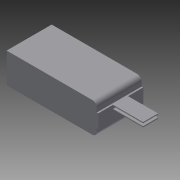
# Autodesk Inventor part: Limit Switch Container
Saved by Autodesk Inventor 2015 (Build 190159000, 159)
## iProperties
Created: 2015-01-10
Part Number: Limit Switch Container
Material: Generic
Document SubType Name: Modeling
Designer: harrykuperstein
Density: 1 g/cm^3
Appearance: Default
Author: harrykuperstein
Autodesk Inventor part; units mm, degrees
ref_plane "YZ Plane" through (0, 0, 0) normal (1, 0, 0) x (0, 1, 0)
ref_plane "XZ Plane" through (0, 0, 0) normal (0, 1, 0) x (-1, 0, 0)
ref_plane "XY Plane" through (0, 0, 0) normal (0, 0, 1) x (1, 0, 0)
sketch "Sketch1" plane through (0, 0, 0) normal (0, 1, 0) x (-1, 0, 0)
  line L0 (0, 0) -> (-30, 0)
  line L1 (-30, 0) -> (-30, -15)
  line L2 (-30, -15) -> (0, -15)
  line L3 (0, -15) -> (0, 0)
  dimension "d0" = 30
  dimension "d1" = 15
  constraints: 8 end point, 2 parallel, 1 horizontal, 1 perpendicular
  measures "d0" distance of L2.end L1.end
  measures "d1" distance of L1.end L0.end
extrude "Extrusion1" add sketch "Sketch1" along normal blind 10
fillet "Fillet1" radius 1.5 1 edges at (30, 10, -7.5)
fillet "Fillet2" radius 1.5 1 edges at (30, 0, -7.5)
fillet "Fillet3" radius 0.5 1 edges at (0, 0, -7.5)
sketch "Sketch2" plane through (30, 8.5, 0) normal (1, 0, 0) x (0, 0, -1)
  line L0 (0, 0) -> (15, 0)
  line L1 (15, 0) -> (0, 0)
  line L2 (15, -7) -> (0, -7) projected
  line L3 (0, -7) -> (0, -6)
  line L4 (0, -6) -> (15, -6)
  line L5 (15, -6) -> (15, -1.3619)
  line L6 (15, -1.3619) -> (0, -1.3619)
  line L7 (0, -1.3619) -> (0, -6)
  point P0 (0, -8.5)
  dimension "d7" = 1
  constraints: 14 end point, 3 horizontal, 2 parallel, 2 vertical, 1 perpendicular
  measures "d7" distance of L3.start L3.end
extrude "Extrusion2" add sketch "Sketch2" along normal blind 0.5
sketch "Sketch3" plane through (30.5, 8.5, 0) normal (1, 0, 0) x (0, 0, -1)
  line L0 (4.9274, -1.3619) -> (9.9274, -1.3619)
  line L1 (0, -1.3619) -> (15, -1.3619) projected
  line L2 (0, 0) -> (15, 0) projected
  line L3 (4.9274, -5.123) -> (9.9274, -5.123)
  line L4 (4.9274, -1.3619) -> (9.9274, -1.3619)
  line L5 (9.9274, -1.3619) -> (9.9274, -1.6824)
  line L6 (9.9274, -1.6824) -> (4.9274, -1.6824)
  line L7 (4.9274, -1.6824) -> (4.9274, -1.3619)
  line L8 (4.9274, -5.123) -> (9.9274, -5.123)
  line L9 (9.9274, -5.123) -> (9.9274, -4.8257)
  line L10 (9.9274, -4.8257) -> (4.9274, -4.8257)
  line L11 (4.9274, -4.8257) -> (4.9274, -5.123)
  point P0 (4.9274, -4.9744)
  point P1 (9.9274, -4.9744)
  point P2 (4.9274, -1.5221)
  point P3 (9.9274, -1.5221)
  dimension "d15" = 5
  dimension "d16" = 5
  constraints: 20 end point, 6 horizontal, 6 parallel, 4 midpoint, 2 perpendicular, 2 point on line, 4 other
  measures "d15" distance of L0.start L0.end
  measures "d16" distance of L3.start L3.end
extrude "Extrusion3" add sketch "Sketch3" along normal blind 10 contours L0 L5 L6 L7
sketch "Sketch5" plane through (30.5, 7.3297, -0.0017) normal (1, 0, 0) x (0, 0, -1)
  line L0 (4.9274, -1.3619) -> (9.9274, -1.3619)
  line L1 (0, -1.3619) -> (15, -1.3619)
  line L2 (0, 0) -> (15, 0)
  line L3 (4.9274, -5.123) -> (9.9274, -5.123)
  line L4 (4.9274, -1.3619) -> (9.9274, -1.3619)
  line L5 (9.9274, -1.3619) -> (9.9274, -1.6824)
  line L6 (9.9274, -1.6824) -> (4.9274, -1.6824)
  line L7 (4.9274, -1.6824) -> (4.9274, -1.3619)
  line L8 (4.9274, -5.123) -> (9.9274, -5.123)
  line L9 (9.9274, -5.123) -> (9.9274, -4.8257)
  line L10 (9.9274, -4.8257) -> (4.9274, -4.8257)
  line L11 (4.9274, -4.8257) -> (4.9274, -5.123)
  point P0 (4.9274, -4.9744)
  point P1 (9.9274, -4.9744)
  point P2 (4.9274, -1.5221)
  point P3 (9.9274, -1.5221)
  dimension "d20" = 5
  dimension "d19" = 5
  constraints: 24 end point, 6 horizontal, 6 parallel, 4 midpoint, 2 perpendicular, 2 point on line, 4 other
  measures "d20" distance of L0.start L0.end
  measures "d19" distance of L3.start L3.end
extrude "Extrusion4" add sketch "Sketch5" along normal blind 10 contours L0 L5 L6 L7
body "Solid1"
